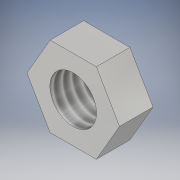
# Autodesk Inventor part: Nut
Saved by Autodesk Inventor 2018 (Build 220112000, 112)
## iProperties
Created: 2018-01-12
Part Number: Nut
Material: Stainless Steel
Document SubType Name: Modeling
Designer: Kyle
Density: 8 g/cm^3
Appearance: Aluminum - Polished
Author: Kyle
Autodesk Inventor part; units mm, degrees
ref_plane "YZ Plane" through (0, 0, 0) normal (1, 0, 0) x (0, 1, 0)
ref_plane "XZ Plane" through (0, 0, 0) normal (0, 1, 0) x (-1, 0, 0)
ref_plane "XY Plane" through (0, 0, 0) normal (0, 0, 1) x (1, 0, 0)
sketch "Sketch1" plane through (0, 0, 0) normal (0, 0, 1) x (1, 0, 0)
  line L0 (-3.1529, 0) -> (-1.5765, 2.7305)
  line L1 (-1.5765, 2.7305) -> (1.5765, 2.7305)
  line L2 (1.5765, 2.7305) -> (3.1529, 0)
  line L3 (3.1529, 0) -> (1.5765, -2.7305)
  line L4 (1.5765, -2.7305) -> (-1.5765, -2.7305)
  line L5 (-1.5765, -2.7305) -> (-3.1529, 0)
  circle A0 centre (0, 0) radius 1.5875
  dimension "d0" = 5.461
  dimension "d1" = 3.175
  constraints: 12 end point, 2 coincident, 1 centre point, 1 horizontal, 13 other
  measures "d0" distance between parallel lines of L4 L1
  measures "d1" diameter of A0
extrude "Extrusion1" add sketch "Sketch1" along normal blind 2.286
thread "Thread1" size "5-40 UNC" class "2B" standard "ANSI Unified Screw Threads" full length
body "Solid1"
